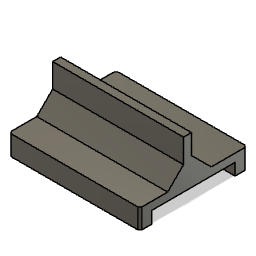
ProMicroBase v3 (Autodesk Fusion 360 design; units mm, degrees)
Autodesk Fusion 360 part; units mm, degrees
note: some values were not read from the file. Set by a fixed rule: which sketch regions a step uses.
sketch "スケッチ1" plane through (0, 0, 0) normal (1, 0, 0) x (0, 0, -1)
  line L0 (0, 2) -> (0, 0)
  line L1 (3, 0) -> (24, 0)
  line L2 (27, 0) -> (27, 2)
  line L3 (27, 2) -> (18, 2)
  line L4 (18, 2) -> (13, 7)
  line L5 (13, 7) -> (13, 12)
  line L6 (13, 12) -> (11, 12)
  line L7 (11, 12) -> (11, 6)
  line L8 (7, 2) -> (0, 2)
  line L9 (11, 6) -> (7, 2)
  line L10 (3, 0) -> (3, -3)
  line L11 (3, -3) -> (0, -3)
  line L12 (0, -3) -> (0, 0)
  line L13 (24, 0) -> (24, -3)
  line L14 (24, -3) -> (27, -3)
  line L15 (27, -3) -> (27, 0)
  point P0 (11, 2)
  dimension "d1" = 4
  dimension "d2" = 4
  dimension "d15" = 27
  dimension "d16" = 3
  dimension "d17" = 3
  dimension "d18" = 3
  dimension "d19" = 3
  constraint coincident L0.end L12.end
  constraint vertical L0
  constraint perpendicular L0 L1
  constraint perpendicular L1 L2
  constraint perpendicular L2 L3
  constraint perpendicular L1 L5
  constraint perpendicular L5 L6
  constraint perpendicular L6 L7
  constraint perpendicular L0 L8
  constraint coincident P0 L7
  constraint coincident P0 L8
  constraint vertical L10
  constraint horizontal L11
  constraint vertical L12
  constraint vertical L13
  constraint horizontal L14
  constraint vertical L15
  measures "d1" distance of P0 L7.end
  measures "d2" distance of P0 L8.start
  measures "d15" distance of L0 L2
  measures "d16" distance of L10 L12
  measures "d17" distance of L2 L13
  measures "d18" distance of L1 L11
  measures "d19" distance of L1 L14
extrude "押し出し1" add sketch "スケッチ1" along normal blind 33
chamfer "面取り1" distance 0.5 angle 45 1 edges at (0, -0.5, -27)
chamfer "面取り2" distance 0.5 angle 45 1 edges at (0, -0.5, 0)
chamfer "面取り3" distance 0.5 angle 45 1 edges at (33, -0.5, -27)
chamfer "面取り4" distance 0.5 angle 45 1 edges at (33, -0.5, 0)
